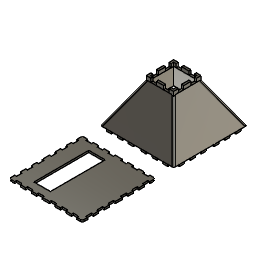
Foot_V2 (Autodesk Fusion 360 design; units mm, degrees)
part number: 2025-04-28-07-17-25-535
part number: 2025-04-28-07-32-23-550
part number: 2025-04-28-07-50-32-250
Autodesk Fusion 360 part; units mm, degrees
sketch "Sketch1" plane through (0, 0, 0) normal (0, 0, 1) x (1, 0, 0) in component "base"
  line L0 (40, -40) -> (-40, -40)
  line L1 (-40, -40) -> (-40, 40)
  line L2 (-40, 40) -> (40, 40)
  line L3 (40, 40) -> (40, -40)
  line L4 (40, -40) -> (-40, 40) construction
  line L5 (-40, -40) -> (40, 40) construction
  dimension "d20" = 80
  dimension "d21" = 80
  constraint horizontal L0
  constraint perpendicular L0 L1
  constraint parallel L0 L2
  constraint parallel L1 L3
  constraint coincident L4 origin
  constraint coincident L5 origin
  measures "d20" distance of L1.end L2.end
  measures "d21" distance of L0.end L1.end
extrude "Extrude1" add sketch "Sketch1" along normal blind 2 makes body 1 in component "base"
sketch "Sketch3" plane through (0, 0, 2) normal (0, 0, 1) x (-1, 0, 0) in component "base"
  line L0 (-40, -40) -> (40, -40)
  line L1 (40, -40) -> (40, 40)
  line L2 (40, 40) -> (-40, 40)
  line L3 (-40, 40) -> (-40, -40)
  line L4 (40, -40) -> (-40, -40)
  line L5 (-40, -40) -> (-40, -38)
  line L6 (-40, -38) -> (40, -38)
  line L7 (40, -38) -> (40, -40)
  line L8 (40, -40) -> (38, -40)
  line L9 (38, -40) -> (38, 40)
  line L10 (38, 40) -> (40, 40)
  line L11 (40, 40) -> (40, -40)
  line L12 (40, -40) -> (34, -40)
  line L13 (34, -40) -> (34, -38)
  line L14 (34, -38) -> (40, -38)
  line L15 (40, -38) -> (40, -40)
  line L16 (28, -38) -> (22, -38)
  line L17 (22, -38) -> (22, -40)
  line L18 (22, -40) -> (28, -40)
  line L19 (28, -40) -> (28, -38)
  line L20 (16, -38) -> (10, -38)
  line L21 (10, -38) -> (10, -40)
  line L22 (10, -40) -> (16, -40)
  line L23 (16, -40) -> (16, -38)
  line L24 (0, -40) -> (3, -40)
  line L25 (3, -40) -> (3, -38)
  line L26 (3, -38) -> (0, -38)
  line L27 (0, -38) -> (0, -40)
  line L28 (40, 3) -> (38, 3)
  line L29 (38, 3) -> (38, -3)
  line L30 (38, -3) -> (40, -3)
  line L31 (40, -3) -> (40, 3)
  line L32 (40, -40) -> (38, -40)
  line L33 (38, -40) -> (38, -34)
  line L34 (38, -34) -> (40, -34)
  line L35 (40, -34) -> (40, -40)
  line L36 (38, -28) -> (40, -28)
  line L37 (40, -28) -> (40, -22)
  line L38 (40, -22) -> (38, -22)
  line L39 (38, -22) -> (38, -28)
  line L40 (38, -16) -> (40, -16)
  line L41 (40, -16) -> (40, -10)
  line L42 (40, -10) -> (38, -10)
  line L43 (38, -10) -> (38, -16)
  line L44 (40, 40) -> (38, 40)
  line L45 (38, 40) -> (38, 34)
  line L46 (38, 34) -> (40, 34)
  line L47 (40, 34) -> (40, 40)
  line L48 (40, 28) -> (38, 28)
  line L49 (38, 28) -> (38, 22)
  line L50 (38, 22) -> (40, 22)
  line L51 (40, 22) -> (40, 28)
  line L52 (40, 16) -> (38, 16)
  line L53 (38, 16) -> (38, 10)
  line L54 (38, 10) -> (40, 10)
  line L55 (40, 10) -> (40, 16)
  line L56 (10, -40) -> (4, -40)
  line L57 (4, -40) -> (4, -38)
  line L58 (4, -38) -> (10, -38)
  line L59 (10, -38) -> (10, -40)
  line L60 (40, -10) -> (38, -10)
  line L61 (38, -10) -> (38, -4)
  line L62 (38, -4) -> (40, -4)
  line L63 (40, -4) -> (40, -10)
  line L64 (38, 10) -> (40, 10)
  line L65 (40, 10) -> (40, 4)
  line L66 (40, 4) -> (38, 4)
  line L67 (38, 4) -> (38, 10)
  line L68 (40, 40) -> (-40, 40)
  line L69 (-40, 40) -> (-40, 38)
  line L70 (-40, 38) -> (40, 38)
  line L71 (40, 38) -> (40, 40)
  line L72 (40, 40) -> (34, 40)
  line L73 (34, 40) -> (34, 38)
  line L74 (34, 38) -> (40, 38)
  line L75 (40, 38) -> (40, 40)
  line L76 (34, 40) -> (28, 40)
  line L77 (28, 40) -> (28, 38)
  line L78 (28, 38) -> (34, 38)
  line L79 (34, 38) -> (34, 40)
  line L80 (28, 40) -> (22, 40)
  line L81 (22, 40) -> (22, 38)
  line L82 (22, 38) -> (28, 38)
  line L83 (28, 38) -> (28, 40)
  line L84 (22, 40) -> (16, 40)
  line L85 (16, 40) -> (16, 38)
  line L86 (16, 38) -> (22, 38)
  line L87 (22, 38) -> (22, 40)
  line L88 (16, 40) -> (10, 40)
  line L89 (10, 40) -> (10, 38)
  line L90 (10, 38) -> (16, 38)
  line L91 (16, 38) -> (16, 40)
  line L92 (10, 40) -> (4, 40)
  line L93 (4, 40) -> (4, 38)
  line L94 (4, 38) -> (10, 38)
  line L95 (10, 38) -> (10, 40)
  dimension "d31" = 80
  dimension "d32" = 2
  dimension "d33" = 2
  dimension "d34" = 80
  dimension "d35" = 80
  dimension "d36" = 2
  constraint horizontal L4
  constraint vertical L5
  constraint horizontal L6
  constraint vertical L7
  constraint coincident L0.end L1.start
  constraint horizontal L8
  constraint vertical L9
  constraint horizontal L10
  constraint vertical L11
  constraint horizontal L12
  constraint vertical L13
  constraint horizontal L14
  constraint vertical L15
  constraint coincident L6 L13.end
  constraint horizontal L16
  constraint vertical L17
  constraint horizontal L18
  constraint vertical L19
  constraint coincident L4 L17.end
  constraint coincident L6 L16.start
  constraint horizontal L20
  constraint vertical L21
  constraint horizontal L22
  constraint vertical L23
  constraint coincident L4 L21.end
  constraint coincident L6 L20.start
  constraint horizontal L24
  constraint vertical L25
  constraint horizontal L26
  constraint vertical L27
  constraint coincident L6 L25.end
  constraint midpoint L0 L24.start
  constraint horizontal L28
  constraint vertical L29
  constraint horizontal L30
  constraint vertical L31
  constraint coincident L9 L29.end
  constraint coincident L11 L28.start
  constraint horizontal L32
  constraint vertical L33
  constraint horizontal L34
  constraint vertical L35
  constraint coincident L9 L33.end
  constraint horizontal L36
  constraint vertical L37
  constraint horizontal L38
  constraint vertical L39
  constraint coincident L1 L37.end
  constraint coincident L9 L36.start
  constraint horizontal L40
  constraint vertical L41
  constraint horizontal L42
  constraint vertical L43
  constraint coincident L11 L41.end
  constraint coincident L9 L40.start
  constraint horizontal L44
  constraint vertical L45
  constraint horizontal L46
  constraint vertical L47
  constraint coincident L9 L45.end
  constraint horizontal L48
  constraint vertical L49
  constraint horizontal L50
  constraint vertical L51
  constraint coincident L9 L49.end
  constraint coincident L11 L48.start
  constraint horizontal L52
  constraint vertical L53
  constraint horizontal L54
  constraint vertical L55
  constraint coincident L9 L53.end
  constraint coincident L11 L52.start
  constraint horizontal L56
  constraint vertical L57
  constraint horizontal L58
  constraint vertical L59
  constraint coincident L6 L57.end
  constraint horizontal L60
  constraint vertical L61
  constraint horizontal L62
  constraint vertical L63
  constraint coincident L9 L61.end
  constraint horizontal L64
  constraint vertical L65
  constraint horizontal L66
  constraint vertical L67
  constraint coincident L11 L65.end
  constraint horizontal L68
  constraint vertical L69
  constraint horizontal L70
  constraint vertical L71
  constraint coincident L1.end L2.start
  constraint horizontal L72
  constraint vertical L73
  constraint horizontal L74
  constraint vertical L75
  constraint coincident L70 L73.end
  constraint horizontal L76
  constraint vertical L77
  constraint horizontal L78
  constraint vertical L79
  constraint coincident L70 L77.end
  constraint horizontal L80
  constraint vertical L81
  constraint horizontal L82
  constraint vertical L83
  constraint coincident L70 L81.end
  constraint horizontal L84
  constraint vertical L85
  constraint horizontal L86
  constraint vertical L87
  constraint coincident L70 L85.end
  constraint horizontal L88
  constraint vertical L89
  constraint horizontal L90
  constraint vertical L91
  constraint coincident L70 L89.end
  constraint horizontal L92
  constraint vertical L93
  constraint horizontal L94
  constraint vertical L95
  constraint coincident L70 L93.end
  measures "d31" distance of L0.end L0.start
  measures "d32" distance of L0.end L6.end
  measures "d33" distance of L0.end L8.end
  measures "d34" distance of L0.end L1.end
  measures "d35" distance of L1.end L2.end
  measures "d36" distance of L1.end L70.end
extrude "Extrude2" cut sketch "Sketch3" against normal blind 2 contours L0 L4 L6 L21 L56 L57 L58 L59 | L2 L68 L70 L89 L92 L93 L94 L95 | L0 L4 L6 L17 L23 | L2 L68 L70 L81 L84 L85 L86 L87 L91 | L0 L4 L6 L13 L19 | L2 L68 L70 L73 L76 L77 L78 L79 L83 | L1 L9 L11 L46 L48 | L1 L9 L11 L34 L36 | L1 L9 L11 L50 L52 | L1 L9 L11 L38 L40 | L1 L9 L11 L54 L64 L65 L66 L67 | L1 L9 L11 L42 L60 L61 L62 L63 bodies 1 in component "base"
mirror "Mirror1" about plane through (0, 0, 0) normal (1, 0, 0) of "Extrude2" in component "base"
sketch "Sketch3 (2)" plane through (0, 0, 0) normal (0, 0, 1) x (1, 0, 0) in component "hat"
  line L0 (40, 40) -> (-40, 40)
  line L1 (-40, 40) -> (-40, -40)
  line L2 (-40, -40) -> (40, -40)
  line L3 (40, -40) -> (40, 40)
  line L4 (40, 40) -> (-40, -40) construction
  line L5 (-40, 40) -> (40, -40) construction
  dimension "d41" = 80
  dimension "d42" = 80
  constraint horizontal L0
  constraint perpendicular L0 L1
  constraint parallel L0 L2
  constraint parallel L1 L3
  constraint coincident L4 origin
  constraint coincident L5 origin
  measures "d41" distance of L1.end L2.end
  measures "d42" distance of L0.end L1.end
extrude "Extrude1'" add sketch "Sketch3 (2)" along normal blind 43.5 separate body makes body 2 in component "hat"
move_body "Move1" bodies 2 to x (1, 0, 0) y (0, 1, 0) z (0, 0, 1) at (0, 0, 2) in component "hat"
ref_plane "WorkPlane1" through (0, -40, 23.75) normal (0, -1, 0) x (1, 0, 0) in component "hat"
ref_plane "WorkPlane2" through (40, 0, 23.75) normal (1, 0, 0) x (0, 1, 0) in component "hat"
sketch "Sketch4" plane through (0, -40, 0) normal (0, -1, 0) x (-1, 0, 0) in component "hat"
  line L0 (-15, -45.5) -> (-40, -2)
  line L1 (-40, -2) -> (-40, -45.5)
  line L2 (-40, -45.5) -> (-15, -45.5)
  line L3 (15, -45.5) -> (40, -45.5)
  line L4 (40, -45.5) -> (40, -2)
  line L5 (40, -2) -> (15, -45.5)
  constraint perpendicular L1 L2
  constraint perpendicular L1 L3
  constraint perpendicular L3 L4
extrude "Extrude2'" cut sketch "Sketch4" against normal blind 80 bodies 2 in component "hat"
sketch "Sketch5" plane through (40, 0, 0) normal (1, 0, 0) x (0, 1, 0) in component "hat"
  line L0 (0, 45.5) -> (-15, 45.5)
  line L1 (0, 45.5) -> (15, 45.5)
  line L2 (-15, 45.5) -> (-40, 45.5)
  line L3 (-40, 45.5) -> (-40, 2)
  line L4 (-40, 2) -> (-15, 45.5)
  line L5 (15, 45.5) -> (40, 2)
  line L6 (40, 2) -> (40, 45.5)
  line L7 (40, 45.5) -> (15, 45.5)
  dimension "d54" = 15
  dimension "d55" = 15
  constraint horizontal L0
  constraint parallel L0 L1
  constraint parallel L0 L2
  constraint perpendicular L2 L3
  constraint perpendicular L1 L6
  constraint perpendicular L6 L7
  measures "d54" distance of L0.start L0.end
  measures "d55" distance of L0.start L1.end
extrude "Extrude3" cut sketch "Sketch5" against normal blind 80 bodies 2 in component "hat"
shell "Shell1" thickness 2 removed faces 2 at (-13.3333, 13.3333, 2) at (-5, 5, 45.5) on bodies 2 in component "hat"
sketch "Sketch6" plane through (0, 0, 2) normal (0, 0, -1) x (1, 0, 0) in component "hat"
  line L0 (-37.6932, 37.6932) -> (37.6932, 37.6932)
  line L1 (37.6932, 37.6932) -> (37.6932, -37.6932)
  line L2 (37.6932, -37.6932) -> (-37.6932, -37.6932)
  line L3 (-37.6932, -37.6932) -> (-37.6932, 37.6932)
  line L4 (40, -40) -> (40, 40)
  line L5 (40, 40) -> (-40, 40)
  line L6 (-40, 40) -> (-40, -40)
  line L7 (-40, -40) -> (40, -40)
  line L8 (33.8, -40) -> (28.2, -40)
  line L9 (28.2, -40) -> (28.2, -38.2)
  line L10 (28.2, -38.2) -> (33.8, -38.2)
  line L11 (33.8, -38.2) -> (33.8, -40)
  line L12 (21.8, -40) -> (16.2, -40)
  line L13 (16.2, -40) -> (16.2, -38.2)
  line L14 (16.2, -38.2) -> (21.8, -38.2)
  line L15 (21.8, -38.2) -> (21.8, -40)
  line L16 (9.8, -40) -> (4.2, -40)
  line L17 (4.2, -40) -> (4.2, -38.2)
  line L18 (4.2, -38.2) -> (9.8, -38.2)
  line L19 (9.8, -38.2) -> (9.8, -40)
  line L20 (38.2, -33.8) -> (40, -33.8)
  line L21 (40, -33.8) -> (40, -28.2)
  line L22 (40, -28.2) -> (38.2, -28.2)
  line L23 (38.2, -28.2) -> (38.2, -33.8)
  line L24 (40, -21.8) -> (38.2, -21.8)
  line L25 (38.2, -21.8) -> (38.2, -16.2)
  line L26 (38.2, -16.2) -> (40, -16.2)
  line L27 (40, -16.2) -> (40, -21.8)
  line L28 (40, -9.8) -> (38.2, -9.8)
  line L29 (38.2, -9.8) -> (38.2, -4.2)
  line L30 (38.2, -4.2) -> (40, -4.2)
  line L31 (40, -4.2) -> (40, -9.8)
  constraint horizontal L8
  constraint vertical L9
  constraint horizontal L10
  constraint vertical L11
  constraint coincident L7 L8.start
  constraint horizontal L12
  constraint vertical L13
  constraint horizontal L14
  constraint vertical L15
  constraint horizontal L16
  constraint vertical L17
  constraint horizontal L18
  constraint vertical L19
  constraint coincident L7 L16.start
  constraint horizontal L20
  constraint vertical L21
  constraint horizontal L22
  constraint vertical L23
  constraint coincident L4 L21.end
  constraint horizontal L24
  constraint vertical L25
  constraint horizontal L26
  constraint vertical L27
  constraint coincident L4 L24.start
  constraint horizontal L28
  constraint vertical L29
  constraint horizontal L30
  constraint vertical L31
  constraint coincident L4 L28.start
extrude "Extrude4" add sketch "Sketch6" along normal blind 2 contours L4 L20 L21 L22 L23 | L7 L8 L9 L10 L11 | L4 L24 L25 L26 L27 | L7 L12 L13 L14 L15 | L4 L28 L29 L30 L31 | L7 L16 L17 L18 L19 bodies 2 in component "hat"
mirror "Mirror1'" about plane through (0, 0, 0) normal (0, 1, 0) of "Extrude4" in component "hat"
mirror "Mirror2" about plane through (0, 0, 0) normal (1, 0, 0) of "Extrude4", "Mirror1'" in component "hat"
sketch "Sketch7" plane through (0, 0, 45.5) normal (0, 0, 1) x (-1, 0, 0) in component "hat"
  line L0 (-12.6932, 12.6932) -> (12.6932, 12.6932)
  line L1 (12.6932, 12.6932) -> (12.6932, -12.6932)
  line L2 (12.6932, -12.6932) -> (-12.6932, -12.6932)
  line L3 (-12.6932, -12.6932) -> (-12.6932, 12.6932)
  line L4 (-15, -15) -> (15, -15)
  line L5 (15, -15) -> (15, 15)
  line L6 (15, 15) -> (-15, 15)
  line L7 (-15, 15) -> (-15, -15)
  line L8 (15, 15) -> (10, 15)
  line L9 (10, 15) -> (10, 12.6932)
  line L10 (10, 12.6932) -> (15, 12.6932)
  line L11 (15, 12.6932) -> (15, 15)
  line L12 (-15, 15) -> (-10, 15)
  line L13 (-10, 15) -> (-10, 12.6932)
  line L14 (-10, 12.6932) -> (-15, 12.6932)
  line L15 (-15, 12.6932) -> (-15, 15)
  line L16 (-10, 15) -> (-4, 15)
  line L17 (-4, 15) -> (-4, 12.6932)
  line L18 (-4, 12.6932) -> (-10, 12.6932)
  line L19 (-10, 12.6932) -> (-10, 15)
  line L20 (10, 15) -> (4, 15)
  line L21 (4, 15) -> (4, 12.6932)
  line L22 (4, 12.6932) -> (10, 12.6932)
  line L23 (10, 12.6932) -> (10, 15)
  line L24 (-15, 15) -> (-12.6932, 15)
  line L25 (-12.6932, 15) -> (-12.6932, 10)
  line L26 (-12.6932, 10) -> (-15, 10)
  line L27 (-15, 10) -> (-15, 15)
  line L28 (-12.6932, 10) -> (-15, 10)
  line L29 (-15, 10) -> (-15, 4)
  line L30 (-15, 4) -> (-12.6932, 4)
  line L31 (-12.6932, 4) -> (-12.6932, 10)
  line L32 (-15, 4) -> (-12.6932, 4)
  line L33 (-12.6932, 4) -> (-12.6932, 0)
  line L34 (-12.6932, 0) -> (-15, 0)
  line L35 (-15, 0) -> (-15, 4)
  dimension "d65" = 5
  dimension "d66" = 5
  dimension "d67" = 6
  dimension "d68" = 6
  dimension "d69" = 5
  constraint horizontal L8
  constraint vertical L9
  constraint horizontal L10
  constraint vertical L11
  constraint coincident L0 L9.end
  constraint coincident L5.end L6.start
  constraint horizontal L12
  constraint vertical L13
  constraint horizontal L14
  constraint vertical L15
  constraint coincident L6.end L7.start
  constraint horizontal L16
  constraint vertical L17
  constraint horizontal L18
  constraint vertical L19
  constraint coincident L0 L17.end
  constraint horizontal L20
  constraint vertical L21
  constraint horizontal L22
  constraint vertical L23
  constraint coincident L0 L21.end
  constraint horizontal L24
  constraint vertical L25
  constraint horizontal L26
  constraint vertical L27
  constraint coincident L3 L25.end
  constraint horizontal L28
  constraint vertical L29
  constraint horizontal L30
  constraint vertical L31
  constraint coincident L7 L29.end
  constraint horizontal L32
  constraint vertical L33
  constraint horizontal L34
  constraint vertical L35
  constraint midpoint L3 L33.end
  measures "d65" distance of L5.end L8.end
  measures "d66" distance of L6.end L12.end
  measures "d67" distance of L12.end L16.end
  measures "d68" distance of L8.end L20.end
  measures "d69" distance of L6.end L26.end
extrude "Extrude5" add sketch "Sketch7" along normal blind 4 contours L0 L6 L12 L13 L14 L19 L25 | L3 L7 L14 L25 L26 L27 L28 | L6 L7 L12 L14 L15 L24 L25 L27 | L0 L6 L17 L21 | L3 L7 L30 L32 L33 L34 L35 bodies 2 in component "hat"
mirror "Mirror3" about plane through (0, 0, 0) normal (0, 1, 0) of "Extrude5" in component "hat"
mirror "Mirror4" about plane through (0, 0, 0) normal (1, 0, 0) of "Extrude5", "Mirror3" in component "hat"
fillet "Fillet1" radius 2 4 edges at (27.5, -27.5, 23.75) (27.5, 27.5, 23.75) (-27.5, -27.5, 23.75) (-27.5, 27.5, 23.75) on bodies 2 in component "hat"
fillet "Fillet1'" radius 2 4 edges at (40, -40, 1) (-40, -40, 1) (-40, 40, 1) (40, 40, 1) on bodies 1 in component "base"
sketch "Sketch4 (2)" plane through (0, 0, 0) normal (0, 0, -1) x (1, 0, 0) in component "base"
  arc A0 (38, -40) -> (40, -38) centre (38, -38) ccw
  line L0 (40, -38) -> (40, -34)
  line L1 (40, -34) -> (38, -34)
  line L2 (38, -34) -> (38, -28)
  line L3 (38, -28) -> (40, -28)
  line L4 (40, -28) -> (40, -22)
  line L5 (40, -22) -> (38, -22)
  line L6 (38, -22) -> (38, -16)
  line L7 (38, -16) -> (40, -16)
  line L8 (40, -16) -> (40, -10)
  line L9 (40, -10) -> (38, -10)
  line L10 (38, -10) -> (38, -4)
  line L11 (38, -4) -> (40, -4)
  line L12 (40, -4) -> (40, 4)
  line L13 (40, 4) -> (38, 4)
  line L14 (38, 4) -> (38, 10)
  line L15 (38, 10) -> (40, 10)
  line L16 (40, 10) -> (40, 16)
  line L17 (40, 16) -> (38, 16)
  line L18 (38, 16) -> (38, 22)
  line L19 (38, 22) -> (40, 22)
  line L20 (40, 22) -> (40, 28)
  line L21 (40, 28) -> (38, 28)
  line L22 (38, 28) -> (38, 34)
  line L23 (38, 34) -> (40, 34)
  line L24 (40, 34) -> (40, 38)
  arc A1 (40, 38) -> (38, 40) centre (38, 38) ccw
  line L25 (38, 40) -> (34, 40)
  line L26 (34, 40) -> (34, 38)
  line L27 (34, 38) -> (28, 38)
  line L28 (28, 38) -> (28, 40)
  line L29 (28, 40) -> (22, 40)
  line L30 (22, 40) -> (22, 38)
  line L31 (22, 38) -> (16, 38)
  line L32 (16, 38) -> (16, 40)
  line L33 (16, 40) -> (10, 40)
  line L34 (10, 40) -> (10, 38)
  line L35 (10, 38) -> (4, 38)
  line L36 (4, 38) -> (4, 40)
  line L37 (4, 40) -> (-4, 40)
  line L38 (-4, 40) -> (-4, 38)
  line L39 (-4, 38) -> (-10, 38)
  line L40 (-10, 38) -> (-10, 40)
  line L41 (-10, 40) -> (-16, 40)
  line L42 (-16, 40) -> (-16, 38)
  line L43 (-16, 38) -> (-22, 38)
  line L44 (-22, 38) -> (-22, 40)
  line L45 (-22, 40) -> (-28, 40)
  line L46 (-28, 40) -> (-28, 38)
  line L47 (-28, 38) -> (-34, 38)
  line L48 (-34, 38) -> (-34, 40)
  line L49 (-34, 40) -> (-38, 40)
  arc A2 (-38, 40) -> (-40, 38) centre (-38, 38) ccw
  line L50 (-40, 38) -> (-40, 34)
  line L51 (-40, 34) -> (-38, 34)
  line L52 (-38, 34) -> (-38, 28)
  line L53 (-38, 28) -> (-40, 28)
  line L54 (-40, 28) -> (-40, 22)
  line L55 (-40, 22) -> (-38, 22)
  line L56 (-38, 22) -> (-38, 16)
  line L57 (-38, 16) -> (-40, 16)
  line L58 (-40, 16) -> (-40, 10)
  line L59 (-40, 10) -> (-38, 10)
  line L60 (-38, 10) -> (-38, 4)
  line L61 (-38, 4) -> (-40, 4)
  line L62 (-40, 4) -> (-40, -4)
  line L63 (-40, -4) -> (-38, -4)
  line L64 (-38, -4) -> (-38, -10)
  line L65 (-38, -10) -> (-40, -10)
  line L66 (-40, -10) -> (-40, -16)
  line L67 (-40, -16) -> (-38, -16)
  line L68 (-38, -16) -> (-38, -22)
  line L69 (-38, -22) -> (-40, -22)
  line L70 (-40, -22) -> (-40, -28)
  line L71 (-40, -28) -> (-38, -28)
  line L72 (-38, -28) -> (-38, -34)
  line L73 (-38, -34) -> (-40, -34)
  line L74 (-40, -34) -> (-40, -38)
  arc A3 (-40, -38) -> (-38, -40) centre (-38, -38) ccw
  line L75 (-38, -40) -> (-34, -40)
  line L76 (-34, -40) -> (-34, -38)
  line L77 (-34, -38) -> (-28, -38)
  line L78 (-28, -38) -> (-28, -40)
  line L79 (-28, -40) -> (-22, -40)
  line L80 (-22, -40) -> (-22, -38)
  line L81 (-22, -38) -> (-16, -38)
  line L82 (-16, -38) -> (-16, -40)
  line L83 (-16, -40) -> (-10, -40)
  line L84 (-10, -40) -> (-10, -38)
  line L85 (-10, -38) -> (-4, -38)
  line L86 (-4, -38) -> (-4, -40)
  line L87 (-4, -40) -> (4, -40)
  line L88 (4, -40) -> (4, -38)
  line L89 (4, -38) -> (10, -38)
  line L90 (10, -38) -> (10, -40)
  line L91 (10, -40) -> (16, -40)
  line L92 (16, -40) -> (16, -38)
  line L93 (16, -38) -> (22, -38)
  line L94 (22, -38) -> (22, -40)
  line L95 (22, -40) -> (28, -40)
  line L96 (28, -40) -> (28, -38)
  line L97 (28, -38) -> (34, -38)
  line L98 (34, -38) -> (34, -40)
  line L99 (34, -40) -> (38, -40)
  line L100 (0, 0) -> (-19, 0)
  line L101 (-23, 0) -> (-5, 0) construction
  line L102 (-5, 0) -> (-5, -30)
  line L103 (-5, -30) -> (-23, -30)
  line L104 (-23, -30) -> (-23, 0)
  line L105 (-5, 0) -> (-23, 0) construction
  line L106 (-23, 0) -> (-23, 30)
  line L107 (-23, 30) -> (-5, 30)
  line L108 (-5, 30) -> (-5, 0)
  constraint coincident L100.start origin
  constraint horizontal L100
  constraint horizontal L101
  constraint vertical L102
  constraint horizontal L103
  constraint vertical L104
  constraint horizontal L105
  constraint vertical L106
  constraint horizontal L107
  constraint vertical L108
extrude "Extrude3'" cut sketch "Sketch4 (2)" against normal blind 2 contours L102 L103 L104 L106 L107 L108 bodies 1 in component "base"
component "base" placed x (1, 0, 0) y (0, 1, 0) z (0, 0, 1) at (0, 0, 0)
component "hat" placed x (1, 0, 0) y (0, 1, 0) z (0, 0, 1) at (0, 0, 0) in component "base"
